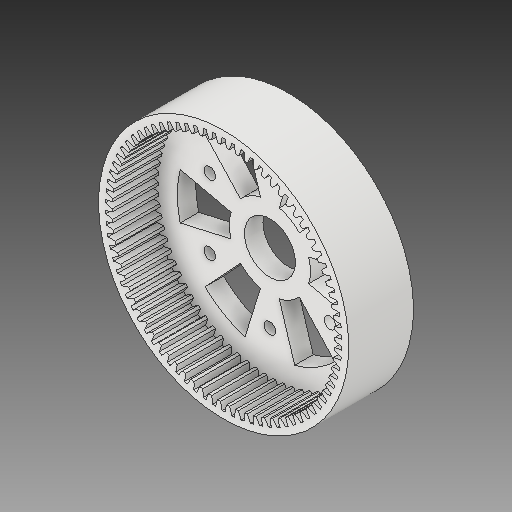
# Autodesk Inventor part: Basespline
Saved by Autodesk Inventor 2017 (Build 210142000, 142)
## iProperties
Created: 2017-07-11
Part Number: Basespline
Material: ABS Plastic
Document SubType Name: Modeling
Designer: zallen
Density: 1.06 g/cm^3
Appearance: CR White
Author: zallen
Autodesk Inventor part; units mm, degrees
ref_plane "YZ Plane" through (0, 0, 0) normal (1, 0, 0) x (0, 1, 0)
ref_plane "XZ Plane" through (0, 0, 0) normal (0, 1, 0) x (-1, 0, 0)
ref_plane "XY Plane" through (0, 0, 0) normal (0, 0, 1) x (1, 0, 0)
sketch "Sketch1" plane through (0, 0, 0) normal (0, 0, 1) x (1, 0, 0)
  circle A0 centre (0, 0) radius 45 construction
  circle A1 centre (0, 0) radius 48 construction
  circle A2 centre (0, 0) radius 48.1 construction
  circle A3 centre (0, 0) radius 51.1
  line L0 (0, 0) -> (73.8871, 0) construction
  circle A4 centre (0, 0) radius 54
  arc A5 (48.0963, -0.6) -> (51.0808, -1.4) centre (53.4515, 13.4115) ccw
  arc A6 (48.0963, 0.6) -> (48.0963, -0.6) centre (68.0873, 0) ccw
  arc A7 (51.0808, 1.4) -> (48.0963, 0.6) centre (53.4515, -13.4115) ccw
  arc A8 (51.0808, -1.4) -> (51.0808, 1.4) centre (0, 0) ccw
  circle A9 centre (0, 0) radius 51.1
  arc A10 (47.9886, 3.2721) -> (51.0278, 2.7148) centre (52.199, 17.669) ccw
  arc A11 (50.8025, 5.5058) -> (47.892, 4.4682) centre (54.3573, -9.0669) ccw
  arc A12 (51.0278, 2.7148) -> (50.8025, 5.5058) centre (0, 0) ccw
  arc A13 (47.892, 4.4682) -> (47.9886, 3.2721) centre (67.8665, 5.4787) ccw
  circle A14 centre (0, 0) radius 51.1
  arc A15 (47.5697, 7.123) -> (50.6439, 6.8121) centre (50.6079, 21.812) ccw
  arc A16 (50.1948, 9.5758) -> (47.3772, 8.3074) centre (54.9107, -4.6636) ccw
  arc A17 (50.6439, 6.8121) -> (50.1948, 9.5758) centre (0, 0) ccw
  arc A18 (47.3772, 8.3074) -> (47.5697, 7.123) centre (67.2055, 10.922) ccw
  circle A19 centre (0, 0) radius 51.1
  arc A20 (46.8423, 10.9276) -> (49.9315, 10.8651) centre (48.6887, 25.8135) ccw
  arc A21 (49.2615, 13.5838) -> (46.5551, 12.0928) centre (55.1079, -0.23) ccw
  arc A22 (49.9315, 10.8651) -> (49.2615, 13.5838) centre (0, 0) ccw
  arc A23 (46.5551, 12.0928) -> (46.8423, 10.9276) centre (66.1088, 16.2943) ccw
  circle A24 centre (0, 0) radius 51.1
  arc A25 (45.8111, 14.6614) -> (48.8954, 14.8477) centre (46.4537, 29.6477) ccw
  arc A26 (48.0087, 17.5036) -> (45.4311, 15.7997) centre (54.9477, 4.2051) ccw
  arc A27 (48.8954, 14.8477) -> (48.0087, 17.5036) centre (0, 0) ccw
  arc A28 (45.4311, 15.7997) -> (45.8111, 14.6614) centre (64.5832, 21.5611) ccw
  circle A29 centre (0, 0) radius 51.1
  arc A30 (44.4827, 18.3001) -> (47.5421, 18.734) centre (43.9174, 33.2895) ccw
  arc A31 (46.4445, 21.3099) -> (44.0124, 19.4041) centre (54.4311, 8.6129) ccw
  arc A32 (47.5421, 18.734) -> (46.4445, 21.3099) centre (0, 0) ccw
  arc A33 (44.0124, 19.4041) -> (44.4827, 18.3001) centre (62.6389, 26.6879) ccw
  circle A34 centre (0, 0) radius 51.1
  arc A35 (42.866, 21.8202) -> (45.8804, 22.4988) centre (41.0963, 36.7154) ccw
  arc A36 (44.5792, 24.9781) -> (42.3083, 22.8827) centre (53.5616, 12.9649) ccw
  arc A37 (45.8804, 22.4988) -> (44.5792, 24.9781) centre (0, 0) ccw
  arc A38 (42.3083, 22.8827) -> (42.866, 21.8202) centre (60.2883, 31.6417) ccw
  circle A39 centre (0, 0) radius 51.1
  arc A40 (40.9712, 25.1987) -> (43.9213, 26.1177) centre (38.0087, 39.9032) ccw
  arc A41 (42.4247, 28.4842) -> (40.3298, 26.2129) centre (52.3446, 17.2327) ccw
  arc A42 (43.9213, 26.1177) -> (42.4247, 28.4842) centre (0, 0) ccw
  arc A43 (40.3298, 26.2129) -> (40.9712, 25.1987) centre (57.5467, 36.3903) ccw
  circle A44 centre (0, 0) radius 51.1
  arc A45 (38.8107, 28.4138) -> (41.6772, 29.5672) centre (34.6746, 42.8323) ccw
  arc A46 (39.9952, 31.8056) -> (38.0898, 29.3731) centre (50.7882, 21.3889) ccw
  arc A47 (41.6772, 29.5672) -> (39.9952, 31.8056) centre (0, 0) ccw
  arc A48 (38.0898, 29.3731) -> (38.8107, 28.4138) centre (54.4319, 40.9029) ccw
  circle A49 centre (0, 0) radius 51.1
  arc A50 (36.3984, 31.4446) -> (39.1629, 32.8249) centre (31.1156, 45.4835) ccw
  arc A51 (37.3062, 34.9208) -> (35.6027, 32.3428) centre (48.9025, 25.4062) ccw
  arc A52 (39.1629, 32.8249) -> (37.3062, 34.9208) centre (0, 0) ccw
  arc A53 (35.6027, 32.3428) -> (36.3984, 31.4446) centre (50.964, 45.1502) ccw
  circle A54 centre (0, 0) radius 51.1
  arc A55 (33.7502, 34.2715) -> (36.3946, 35.8698) centre (27.3547, 47.8398) ccw
  arc A56 (34.3752, 37.8094) -> (32.8847, 35.1028) centre (46.6995, 29.2589) ccw
  arc A57 (36.3946, 35.8698) -> (34.3752, 37.8094) centre (0, 0) ccw
  arc A58 (32.8847, 35.1028) -> (33.7502, 34.2715) centre (47.1657, 49.1047) ccw
  circle A59 centre (0, 0) radius 51.1
  arc A60 (30.883, 36.8761) -> (33.3903, 38.682) centre (23.4165, 49.8858) ccw
  arc A61 (31.2214, 40.4529) -> (29.9535, 37.6351) centre (44.1937, 32.9218) ccw
  arc A62 (33.3903, 38.682) -> (31.2214, 40.4529) centre (0, 0) ccw
  arc A63 (29.9535, 37.6351) -> (30.883, 36.8761) centre (43.0615, 52.7407) ccw
  circle A64 centre (0, 0) radius 51.1
  arc A65 (27.8156, 39.2416) -> (30.1694, 41.2434) centre (19.3265, 51.6083) ccw
  arc A66 (27.865, 42.834) -> (26.828, 39.9233) centre (41.4013, 36.3711) ccw
  arc A67 (30.1694, 41.2434) -> (27.865, 42.834) centre (0, 0) ccw
  arc A68 (26.828, 39.9233) -> (27.8156, 39.2416) centre (38.678, 56.0347) ccw
  circle A69 centre (0, 0) radius 51.1
  arc A70 (24.5677, 41.3526) -> (26.7528, 43.5373) centre (15.1111, 52.9961) ccw
  arc A71 (24.328, 44.9373) -> (23.5285, 41.9526) centre (38.3404, 39.5846) ccw
  arc A72 (26.7528, 43.5373) -> (24.328, 44.9373) centre (0, 0) ccw
  arc A73 (23.5285, 41.9526) -> (24.5677, 41.3526) centre (34.0436, 58.9653) ccw
  circle A74 centre (0, 0) radius 51.1
  arc A75 (21.1606, 43.1954) -> (23.1628, 45.5488) centre (10.7976, 54.0402) ccw
  arc A76 (20.6331, 46.7492) -> (20.0764, 43.7098) centre (35.0309, 42.5414) ccw
  arc A77 (23.1628, 45.5488) -> (20.6331, 46.7492) centre (0, 0) ccw
  arc A78 (20.0764, 43.7098) -> (21.1606, 43.1954) centre (29.1885, 61.5135) ccw
  circle A79 centre (0, 0) radius 51.1
  arc A80 (17.6162, 44.758) -> (19.4225, 47.2649) centre (6.4142, 54.7338) ccw
  arc A81 (16.8045, 48.2578) -> (16.4942, 45.1835) centre (31.4941, 45.2222) ccw
  arc A82 (19.4225, 47.2649) -> (16.8045, 48.2578) centre (0, 0) ccw
  arc A83 (16.4942, 45.1835) -> (17.6162, 44.758) centre (24.1441, 63.6627) ccw
  circle A84 centre (0, 0) radius 51.1
  arc A85 (13.9575, 46.0304) -> (15.5563, 48.6745) centre (1.9892, 55.0724) ccw
  arc A86 (12.8669, 49.4536) -> (12.8049, 46.3643) centre (27.7531, 47.6098) ccw
  arc A87 (15.5563, 48.6745) -> (12.8669, 49.4536) centre (0, 0) ccw
  arc A88 (12.8049, 46.3643) -> (13.9575, 46.0304) centre (18.9431, 65.399) ccw
  circle A89 centre (0, 0) radius 51.1
  arc A90 (10.2084, 47.0042) -> (11.5892, 49.7685) centre (-2.4488, 55.0539) ccw
  arc A91 (8.8458, 50.3285) -> (9.0326, 47.2443) centre (23.8321, 49.6886) ccw
  arc A92 (11.5892, 49.7685) -> (8.8458, 50.3285) centre (0, 0) ccw
  arc A93 (9.0326, 47.2443) -> (10.2084, 47.0042) centre (13.6192, 66.7113) ccw
  circle A94 centre (0, 0) radius 51.1
  arc A95 (6.393, 47.6733) -> (7.5469, 50.5396) centre (-6.8708, 54.6783) ccw
  arc A96 (4.7673, 50.8771) -> (5.2017, 47.8179) centre (19.7566, 51.4452) ccw
  arc A97 (7.5469, 50.5396) -> (4.7673, 50.8771) centre (0, 0) ccw
  arc A98 (5.2017, 47.8179) -> (6.393, 47.6733) centre (8.207, 67.5908) ccw
  circle A99 centre (0, 0) radius 51.1
  arc A100 (2.5362, 48.0331) -> (3.4557, 50.983) centre (-11.2483, 53.9482) ccw
  arc A101 (0.658, 51.0958) -> (1.3371, 48.0814) centre (15.5529, 52.8681) ccw
  arc A102 (3.4557, 50.983) -> (0.658, 51.0958) centre (0, 0) ccw
  arc A103 (1.3371, 48.0814) -> (2.5362, 48.0331) centre (2.7416, 68.032) ccw
  circle A104 centre (0, 0) radius 51.1
  arc A105 (-1.3371, 48.0814) -> (-0.658, 51.0958) centre (-15.5529, 52.8681) ccw
  arc A106 (-3.4557, 50.983) -> (-2.5362, 48.0331) centre (11.2483, 53.9482) ccw
  arc A107 (-0.658, 51.0958) -> (-3.4557, 50.983) centre (0, 0) ccw
  arc A108 (-2.5362, 48.0331) -> (-1.3371, 48.0814) centre (-2.7416, 68.032) ccw
  circle A109 centre (0, 0) radius 51.1
  arc A110 (-5.2017, 47.8179) -> (-4.7673, 50.8771) centre (-19.7566, 51.4452) ccw
  arc A111 (-7.5469, 50.5396) -> (-6.393, 47.6733) centre (6.8708, 54.6783) ccw
  arc A112 (-4.7673, 50.8771) -> (-7.5469, 50.5396) centre (0, 0) ccw
  arc A113 (-6.393, 47.6733) -> (-5.2017, 47.8179) centre (-8.207, 67.5908) ccw
  circle A114 centre (0, 0) radius 51.1
  arc A115 (-9.0326, 47.2443) -> (-8.8458, 50.3285) centre (-23.8321, 49.6886) ccw
  arc A116 (-11.5892, 49.7685) -> (-10.2084, 47.0042) centre (2.4488, 55.0539) ccw
  arc A117 (-8.8458, 50.3285) -> (-11.5892, 49.7685) centre (0, 0) ccw
  arc A118 (-10.2084, 47.0042) -> (-9.0326, 47.2443) centre (-13.6192, 66.7113) ccw
  circle A119 centre (0, 0) radius 51.1
  arc A120 (-12.8049, 46.3643) -> (-12.8669, 49.4536) centre (-27.7531, 47.6098) ccw
  arc A121 (-15.5563, 48.6745) -> (-13.9575, 46.0304) centre (-1.9892, 55.0724) ccw
  arc A122 (-12.8669, 49.4536) -> (-15.5563, 48.6745) centre (0, 0) ccw
  arc A123 (-13.9575, 46.0304) -> (-12.8049, 46.3643) centre (-18.9431, 65.399) ccw
  circle A124 centre (0, 0) radius 51.1
  arc A125 (-16.4942, 45.1835) -> (-16.8045, 48.2578) centre (-31.4941, 45.2222) ccw
  arc A126 (-19.4225, 47.2649) -> (-17.6162, 44.758) centre (-6.4142, 54.7338) ccw
  arc A127 (-16.8045, 48.2578) -> (-19.4225, 47.2649) centre (0, 0) ccw
  arc A128 (-17.6162, 44.758) -> (-16.4942, 45.1835) centre (-24.1441, 63.6627) ccw
  circle A129 centre (0, 0) radius 51.1
  arc A130 (-20.0764, 43.7098) -> (-20.6331, 46.7492) centre (-35.0309, 42.5414) ccw
  arc A131 (-23.1628, 45.5488) -> (-21.1606, 43.1954) centre (-10.7976, 54.0402) ccw
  arc A132 (-20.6331, 46.7492) -> (-23.1628, 45.5488) centre (0, 0) ccw
  arc A133 (-21.1606, 43.1954) -> (-20.0764, 43.7098) centre (-29.1885, 61.5135) ccw
  circle A134 centre (0, 0) radius 51.1
  arc A135 (-23.5285, 41.9526) -> (-24.328, 44.9373) centre (-38.3404, 39.5846) ccw
  arc A136 (-26.7528, 43.5373) -> (-24.5677, 41.3526) centre (-15.1111, 52.9961) ccw
  arc A137 (-24.328, 44.9373) -> (-26.7528, 43.5373) centre (0, 0) ccw
  arc A138 (-24.5677, 41.3526) -> (-23.5285, 41.9526) centre (-34.0436, 58.9653) ccw
  circle A139 centre (0, 0) radius 51.1
  arc A140 (-26.828, 39.9233) -> (-27.865, 42.834) centre (-41.4013, 36.3711) ccw
  arc A141 (-30.1694, 41.2434) -> (-27.8156, 39.2416) centre (-19.3265, 51.6083) ccw
  arc A142 (-27.865, 42.834) -> (-30.1694, 41.2434) centre (0, 0) ccw
  arc A143 (-27.8156, 39.2416) -> (-26.828, 39.9233) centre (-38.678, 56.0347) ccw
  circle A144 centre (0, 0) radius 51.1
  arc A145 (-29.9535, 37.6351) -> (-31.2214, 40.4529) centre (-44.1937, 32.9218) ccw
  arc A146 (-33.3903, 38.682) -> (-30.883, 36.8761) centre (-23.4165, 49.8858) ccw
  arc A147 (-31.2214, 40.4529) -> (-33.3903, 38.682) centre (0, 0) ccw
  arc A148 (-30.883, 36.8761) -> (-29.9535, 37.6351) centre (-43.0615, 52.7407) ccw
  circle A149 centre (0, 0) radius 51.1
  arc A150 (-32.8847, 35.1028) -> (-34.3752, 37.8094) centre (-46.6995, 29.2589) ccw
  arc A151 (-36.3946, 35.8698) -> (-33.7502, 34.2715) centre (-27.3547, 47.8398) ccw
  arc A152 (-34.3752, 37.8094) -> (-36.3946, 35.8698) centre (0, 0) ccw
  arc A153 (-33.7502, 34.2715) -> (-32.8847, 35.1028) centre (-47.1657, 49.1047) ccw
  circle A154 centre (0, 0) radius 51.1
  arc A155 (-35.6027, 32.3428) -> (-37.3062, 34.9208) centre (-48.9025, 25.4062) ccw
  arc A156 (-39.1629, 32.8249) -> (-36.3984, 31.4446) centre (-31.1156, 45.4835) ccw
  arc A157 (-37.3062, 34.9208) -> (-39.1629, 32.8249) centre (0, 0) ccw
  arc A158 (-36.3984, 31.4446) -> (-35.6027, 32.3428) centre (-50.964, 45.1502) ccw
  circle A159 centre (0, 0) radius 51.1
  arc A160 (-38.0898, 29.3731) -> (-39.9952, 31.8056) centre (-50.7882, 21.3889) ccw
  arc A161 (-41.6772, 29.5672) -> (-38.8107, 28.4138) centre (-34.6746, 42.8323) ccw
  arc A162 (-39.9952, 31.8056) -> (-41.6772, 29.5672) centre (0, 0) ccw
  arc A163 (-38.8107, 28.4138) -> (-38.0898, 29.3731) centre (-54.4319, 40.9029) ccw
  circle A164 centre (0, 0) radius 51.1
  arc A165 (-40.3298, 26.2129) -> (-42.4247, 28.4842) centre (-52.3446, 17.2327) ccw
  arc A166 (-43.9213, 26.1177) -> (-40.9712, 25.1987) centre (-38.0087, 39.9032) ccw
  arc A167 (-42.4247, 28.4842) -> (-43.9213, 26.1177) centre (0, 0) ccw
  arc A168 (-40.9712, 25.1987) -> (-40.3298, 26.2129) centre (-57.5467, 36.3903) ccw
  circle A169 centre (0, 0) radius 51.1
  arc A170 (-42.3083, 22.8827) -> (-44.5792, 24.9781) centre (-53.5616, 12.9649) ccw
  arc A171 (-45.8804, 22.4988) -> (-42.866, 21.8202) centre (-41.0963, 36.7154) ccw
  arc A172 (-44.5792, 24.9781) -> (-45.8804, 22.4988) centre (0, 0) ccw
  arc A173 (-42.866, 21.8202) -> (-42.3083, 22.8827) centre (-60.2883, 31.6417) ccw
  circle A174 centre (0, 0) radius 51.1
  arc A175 (-44.0124, 19.4041) -> (-46.4445, 21.3099) centre (-54.4311, 8.6129) ccw
  arc A176 (-47.5421, 18.734) -> (-44.4827, 18.3001) centre (-43.9174, 33.2895) ccw
  arc A177 (-46.4445, 21.3099) -> (-47.5421, 18.734) centre (0, 0) ccw
  arc A178 (-44.4827, 18.3001) -> (-44.0124, 19.4041) centre (-62.6389, 26.6879) ccw
  circle A179 centre (0, 0) radius 51.1
  arc A180 (-45.4311, 15.7997) -> (-48.0087, 17.5036) centre (-54.9477, 4.2051) ccw
  arc A181 (-48.8954, 14.8477) -> (-45.8111, 14.6614) centre (-46.4537, 29.6477) ccw
  arc A182 (-48.0087, 17.5036) -> (-48.8954, 14.8477) centre (0, 0) ccw
  arc A183 (-45.8111, 14.6614) -> (-45.4311, 15.7997) centre (-64.5832, 21.5611) ccw
  circle A184 centre (0, 0) radius 51.1
  arc A185 (-46.5551, 12.0928) -> (-49.2615, 13.5838) centre (-55.1079, -0.23) ccw
  arc A186 (-49.9315, 10.8651) -> (-46.8423, 10.9276) centre (-48.6887, 25.8135) ccw
  arc A187 (-49.2615, 13.5838) -> (-49.9315, 10.8651) centre (0, 0) ccw
  arc A188 (-46.8423, 10.9276) -> (-46.5551, 12.0928) centre (-66.1088, 16.2943) ccw
  circle A189 centre (0, 0) radius 51.1
  arc A190 (-47.3772, 8.3074) -> (-50.1948, 9.5758) centre (-54.9107, -4.6636) ccw
  arc A191 (-50.6439, 6.8121) -> (-47.5697, 7.123) centre (-50.6079, 21.812) ccw
  arc A192 (-50.1948, 9.5758) -> (-50.6439, 6.8121) centre (0, 0) ccw
  arc A193 (-47.5697, 7.123) -> (-47.3772, 8.3074) centre (-67.2055, 10.922) ccw
  circle A194 centre (0, 0) radius 51.1
  arc A195 (-47.892, 4.4682) -> (-50.8025, 5.5058) centre (-54.3573, -9.0669) ccw
  arc A196 (-51.0278, 2.7148) -> (-47.9886, 3.2721) centre (-52.199, 17.669) ccw
  arc A197 (-50.8025, 5.5058) -> (-51.0278, 2.7148) centre (0, 0) ccw
  arc A198 (-47.9886, 3.2721) -> (-47.892, 4.4682) centre (-67.8665, 5.4787) ccw
  circle A199 centre (0, 0) radius 51.1
  arc A200 (-48.0963, 0.6) -> (-51.0808, 1.4) centre (-53.4515, -13.4115) ccw
  arc A201 (-51.0808, -1.4) -> (-48.0963, -0.6) centre (-53.4515, 13.4115) ccw
  arc A202 (-51.0808, 1.4) -> (-51.0808, -1.4) centre (0, 0) ccw
  arc A203 (-48.0963, -0.6) -> (-48.0963, 0.6) centre (-68.0873, 0) ccw
  circle A204 centre (0, 0) radius 51.1
  arc A205 (-47.9886, -3.2721) -> (-51.0278, -2.7148) centre (-52.199, -17.669) ccw
  arc A206 (-50.8025, -5.5058) -> (-47.892, -4.4682) centre (-54.3573, 9.0669) ccw
  arc A207 (-51.0278, -2.7148) -> (-50.8025, -5.5058) centre (0, 0) ccw
  arc A208 (-47.892, -4.4682) -> (-47.9886, -3.2721) centre (-67.8665, -5.4787) ccw
  circle A209 centre (0, 0) radius 51.1
  arc A210 (-47.5697, -7.123) -> (-50.6439, -6.8121) centre (-50.6079, -21.812) ccw
  arc A211 (-50.1948, -9.5758) -> (-47.3772, -8.3074) centre (-54.9107, 4.6636) ccw
  arc A212 (-50.6439, -6.8121) -> (-50.1948, -9.5758) centre (0, 0) ccw
  arc A213 (-47.3772, -8.3074) -> (-47.5697, -7.123) centre (-67.2055, -10.922) ccw
  circle A214 centre (0, 0) radius 51.1
  arc A215 (-46.8423, -10.9276) -> (-49.9315, -10.8651) centre (-48.6887, -25.8135) ccw
  arc A216 (-49.2615, -13.5838) -> (-46.5551, -12.0928) centre (-55.1079, 0.23) ccw
  arc A217 (-49.9315, -10.8651) -> (-49.2615, -13.5838) centre (0, 0) ccw
  arc A218 (-46.5551, -12.0928) -> (-46.8423, -10.9276) centre (-66.1088, -16.2943) ccw
  circle A219 centre (0, 0) radius 51.1
  arc A220 (-45.8111, -14.6614) -> (-48.8954, -14.8477) centre (-46.4537, -29.6477) ccw
  arc A221 (-48.0087, -17.5036) -> (-45.4311, -15.7997) centre (-54.9477, -4.2051) ccw
  arc A222 (-48.8954, -14.8477) -> (-48.0087, -17.5036) centre (0, 0) ccw
  arc A223 (-45.4311, -15.7997) -> (-45.8111, -14.6614) centre (-64.5832, -21.5611) ccw
  circle A224 centre (0, 0) radius 51.1
  arc A225 (-44.4827, -18.3001) -> (-47.5421, -18.734) centre (-43.9174, -33.2895) ccw
  arc A226 (-46.4445, -21.3099) -> (-44.0124, -19.4041) centre (-54.4311, -8.6129) ccw
  arc A227 (-47.5421, -18.734) -> (-46.4445, -21.3099) centre (0, 0) ccw
  arc A228 (-44.0124, -19.4041) -> (-44.4827, -18.3001) centre (-62.6389, -26.6879) ccw
  circle A229 centre (0, 0) radius 51.1
  arc A230 (-42.866, -21.8202) -> (-45.8804, -22.4988) centre (-41.0963, -36.7154) ccw
  arc A231 (-44.5792, -24.9781) -> (-42.3083, -22.8827) centre (-53.5616, -12.9649) ccw
  arc A232 (-45.8804, -22.4988) -> (-44.5792, -24.9781) centre (0, 0) ccw
  arc A233 (-42.3083, -22.8827) -> (-42.866, -21.8202) centre (-60.2883, -31.6417) ccw
  circle A234 centre (0, 0) radius 51.1
  arc A235 (-40.9712, -25.1987) -> (-43.9213, -26.1177) centre (-38.0087, -39.9032) ccw
  arc A236 (-42.4247, -28.4842) -> (-40.3298, -26.2129) centre (-52.3446, -17.2327) ccw
  arc A237 (-43.9213, -26.1177) -> (-42.4247, -28.4842) centre (0, 0) ccw
  arc A238 (-40.3298, -26.2129) -> (-40.9712, -25.1987) centre (-57.5467, -36.3903) ccw
  circle A239 centre (0, 0) radius 51.1
  arc A240 (-38.8107, -28.4138) -> (-41.6772, -29.5672) centre (-34.6746, -42.8323) ccw
  arc A241 (-39.9952, -31.8056) -> (-38.0898, -29.3731) centre (-50.7882, -21.3889) ccw
  arc A242 (-41.6772, -29.5672) -> (-39.9952, -31.8056) centre (0, 0) ccw
  arc A243 (-38.0898, -29.3731) -> (-38.8107, -28.4138) centre (-54.4319, -40.9029) ccw
  circle A244 centre (0, 0) radius 51.1
  arc A245 (-36.3984, -31.4446) -> (-39.1629, -32.8249) centre (-31.1156, -45.4835) ccw
  arc A246 (-37.3062, -34.9208) -> (-35.6027, -32.3428) centre (-48.9025, -25.4062) ccw
  arc A247 (-39.1629, -32.8249) -> (-37.3062, -34.9208) centre (0, 0) ccw
  arc A248 (-35.6027, -32.3428) -> (-36.3984, -31.4446) centre (-50.964, -45.1502) ccw
  circle A249 centre (0, 0) radius 51.1
  arc A250 (-33.7502, -34.2715) -> (-36.3946, -35.8698) centre (-27.3547, -47.8398) ccw
  arc A251 (-34.3752, -37.8094) -> (-32.8847, -35.1028) centre (-46.6995, -29.2589) ccw
  arc A252 (-36.3946, -35.8698) -> (-34.3752, -37.8094) centre (0, 0) ccw
  arc A253 (-32.8847, -35.1028) -> (-33.7502, -34.2715) centre (-47.1657, -49.1047) ccw
  circle A254 centre (0, 0) radius 51.1
  arc A255 (-30.883, -36.8761) -> (-33.3903, -38.682) centre (-23.4165, -49.8858) ccw
  arc A256 (-31.2214, -40.4529) -> (-29.9535, -37.6351) centre (-44.1937, -32.9218) ccw
  arc A257 (-33.3903, -38.682) -> (-31.2214, -40.4529) centre (0, 0) ccw
  arc A258 (-29.9535, -37.6351) -> (-30.883, -36.8761) centre (-43.0615, -52.7407) ccw
  circle A259 centre (0, 0) radius 51.1
  arc A260 (-27.8156, -39.2416) -> (-30.1694, -41.2434) centre (-19.3265, -51.6083) ccw
  arc A261 (-27.865, -42.834) -> (-26.828, -39.9233) centre (-41.4013, -36.3711) ccw
  arc A262 (-30.1694, -41.2434) -> (-27.865, -42.834) centre (0, 0) ccw
  arc A263 (-26.828, -39.9233) -> (-27.8156, -39.2416) centre (-38.678, -56.0347) ccw
  circle A264 centre (0, 0) radius 51.1
  arc A265 (-24.5677, -41.3526) -> (-26.7528, -43.5373) centre (-15.1111, -52.9961) ccw
  arc A266 (-24.328, -44.9373) -> (-23.5285, -41.9526) centre (-38.3404, -39.5846) ccw
  arc A267 (-26.7528, -43.5373) -> (-24.328, -44.9373) centre (0, 0) ccw
  arc A268 (-23.5285, -41.9526) -> (-24.5677, -41.3526) centre (-34.0436, -58.9653) ccw
  circle A269 centre (0, 0) radius 51.1
  arc A270 (-21.1606, -43.1954) -> (-23.1628, -45.5488) centre (-10.7976, -54.0402) ccw
  arc A271 (-20.6331, -46.7492) -> (-20.0764, -43.7098) centre (-35.0309, -42.5414) ccw
  arc A272 (-23.1628, -45.5488) -> (-20.6331, -46.7492) centre (0, 0) ccw
  arc A273 (-20.0764, -43.7098) -> (-21.1606, -43.1954) centre (-29.1885, -61.5135) ccw
  circle A274 centre (0, 0) radius 51.1
  arc A275 (-17.6162, -44.758) -> (-19.4225, -47.2649) centre (-6.4142, -54.7338) ccw
  arc A276 (-16.8045, -48.2578) -> (-16.4942, -45.1835) centre (-31.4941, -45.2222) ccw
  arc A277 (-19.4225, -47.2649) -> (-16.8045, -48.2578) centre (0, 0) ccw
  arc A278 (-16.4942, -45.1835) -> (-17.6162, -44.758) centre (-24.1441, -63.6627) ccw
  circle A279 centre (0, 0) radius 51.1
  arc A280 (-13.9575, -46.0304) -> (-15.5563, -48.6745) centre (-1.9892, -55.0724) ccw
  arc A281 (-12.8669, -49.4536) -> (-12.8049, -46.3643) centre (-27.7531, -47.6098) ccw
  arc A282 (-15.5563, -48.6745) -> (-12.8669, -49.4536) centre (0, 0) ccw
  arc A283 (-12.8049, -46.3643) -> (-13.9575, -46.0304) centre (-18.9431, -65.399) ccw
  circle A284 centre (0, 0) radius 51.1
  arc A285 (-10.2084, -47.0042) -> (-11.5892, -49.7685) centre (2.4488, -55.0539) ccw
  arc A286 (-8.8458, -50.3285) -> (-9.0326, -47.2443) centre (-23.8321, -49.6886) ccw
  arc A287 (-11.5892, -49.7685) -> (-8.8458, -50.3285) centre (0, 0) ccw
  arc A288 (-9.0326, -47.2443) -> (-10.2084, -47.0042) centre (-13.6192, -66.7113) ccw
  circle A289 centre (0, 0) radius 51.1
  arc A290 (-6.393, -47.6733) -> (-7.5469, -50.5396) centre (6.8708, -54.6783) ccw
  arc A291 (-4.7673, -50.8771) -> (-5.2017, -47.8179) centre (-19.7566, -51.4452) ccw
  arc A292 (-7.5469, -50.5396) -> (-4.7673, -50.8771) centre (0, 0) ccw
  arc A293 (-5.2017, -47.8179) -> (-6.393, -47.6733) centre (-8.207, -67.5908) ccw
  circle A294 centre (0, 0) radius 51.1
  arc A295 (-2.5362, -48.0331) -> (-3.4557, -50.983) centre (11.2483, -53.9482) ccw
  arc A296 (-0.658, -51.0958) -> (-1.3371, -48.0814) centre (-15.5529, -52.8681) ccw
  arc A297 (-3.4557, -50.983) -> (-0.658, -51.0958) centre (0, 0) ccw
  arc A298 (-1.3371, -48.0814) -> (-2.5362, -48.0331) centre (-2.7416, -68.032) ccw
  circle A299 centre (0, 0) radius 51.1
  arc A300 (1.3371, -48.0814) -> (0.658, -51.0958) centre (15.5529, -52.8681) ccw
  arc A301 (3.4557, -50.983) -> (2.5362, -48.0331) centre (-11.2483, -53.9482) ccw
  arc A302 (0.658, -51.0958) -> (3.4557, -50.983) centre (0, 0) ccw
  arc A303 (2.5362, -48.0331) -> (1.3371, -48.0814) centre (2.7416, -68.032) ccw
  circle A304 centre (0, 0) radius 51.1
  arc A305 (5.2017, -47.8179) -> (4.7673, -50.8771) centre (19.7566, -51.4452) ccw
  arc A306 (7.5469, -50.5396) -> (6.393, -47.6733) centre (-6.8708, -54.6783) ccw
  arc A307 (4.7673, -50.8771) -> (7.5469, -50.5396) centre (0, 0) ccw
  arc A308 (6.393, -47.6733) -> (5.2017, -47.8179) centre (8.207, -67.5908) ccw
  circle A309 centre (0, 0) radius 51.1
  arc A310 (9.0326, -47.2443) -> (8.8458, -50.3285) centre (23.8321, -49.6886) ccw
  arc A311 (11.5892, -49.7685) -> (10.2084, -47.0042) centre (-2.4488, -55.0539) ccw
  arc A312 (8.8458, -50.3285) -> (11.5892, -49.7685) centre (0, 0) ccw
  arc A313 (10.2084, -47.0042) -> (9.0326, -47.2443) centre (13.6192, -66.7113) ccw
  circle A314 centre (0, 0) radius 51.1
  arc A315 (12.8049, -46.3643) -> (12.8669, -49.4536) centre (27.7531, -47.6098) ccw
  arc A316 (15.5563, -48.6745) -> (13.9575, -46.0304) centre (1.9892, -55.0724) ccw
  arc A317 (12.8669, -49.4536) -> (15.5563, -48.6745) centre (0, 0) ccw
  arc A318 (13.9575, -46.0304) -> (12.8049, -46.3643) centre (18.9431, -65.399) ccw
  circle A319 centre (0, 0) radius 51.1
  arc A320 (16.4942, -45.1835) -> (16.8045, -48.2578) centre (31.4941, -45.2222) ccw
  arc A321 (19.4225, -47.2649) -> (17.6162, -44.758) centre (6.4142, -54.7338) ccw
  arc A322 (16.8045, -48.2578) -> (19.4225, -47.2649) centre (0, 0) ccw
  arc A323 (17.6162, -44.758) -> (16.4942, -45.1835) centre (24.1441, -63.6627) ccw
  circle A324 centre (0, 0) radius 51.1
  arc A325 (20.0764, -43.7098) -> (20.6331, -46.7492) centre (35.0309, -42.5414) ccw
  arc A326 (23.1628, -45.5488) -> (21.1606, -43.1954) centre (10.7976, -54.0402) ccw
  arc A327 (20.6331, -46.7492) -> (23.1628, -45.5488) centre (0, 0) ccw
  arc A328 (21.1606, -43.1954) -> (20.0764, -43.7098) centre (29.1885, -61.5135) ccw
  circle A329 centre (0, 0) radius 51.1
  arc A330 (23.5285, -41.9526) -> (24.328, -44.9373) centre (38.3404, -39.5846) ccw
  arc A331 (26.7528, -43.5373) -> (24.5677, -41.3526) centre (15.1111, -52.9961) ccw
  arc A332 (24.328, -44.9373) -> (26.7528, -43.5373) centre (0, 0) ccw
  arc A333 (24.5677, -41.3526) -> (23.5285, -41.9526) centre (34.0436, -58.9653) ccw
  circle A334 centre (0, 0) radius 51.1
  arc A335 (26.828, -39.9233) -> (27.865, -42.834) centre (41.4013, -36.3711) ccw
  arc A336 (30.1694, -41.2434) -> (27.8156, -39.2416) centre (19.3265, -51.6083) ccw
  arc A337 (27.865, -42.834) -> (30.1694, -41.2434) centre (0, 0) ccw
  arc A338 (27.8156, -39.2416) -> (26.828, -39.9233) centre (38.678, -56.0347) ccw
  circle A339 centre (0, 0) radius 51.1
  arc A340 (29.9535, -37.6351) -> (31.2214, -40.4529) centre (44.1937, -32.9218) ccw
  arc A341 (33.3903, -38.682) -> (30.883, -36.8761) centre (23.4165, -49.8858) ccw
  arc A342 (31.2214, -40.4529) -> (33.3903, -38.682) centre (0, 0) ccw
  arc A343 (30.883, -36.8761) -> (29.9535, -37.6351) centre (43.0615, -52.7407) ccw
  circle A344 centre (0, 0) radius 51.1
  arc A345 (32.8847, -35.1028) -> (34.3752, -37.8094) centre (46.6995, -29.2589) ccw
  arc A346 (36.3946, -35.8698) -> (33.7502, -34.2715) centre (27.3547, -47.8398) ccw
  arc A347 (34.3752, -37.8094) -> (36.3946, -35.8698) centre (0, 0) ccw
  arc A348 (33.7502, -34.2715) -> (32.8847, -35.1028) centre (47.1657, -49.1047) ccw
  circle A349 centre (0, 0) radius 51.1
  arc A350 (35.6027, -32.3428) -> (37.3062, -34.9208) centre (48.9025, -25.4062) ccw
  arc A351 (39.1629, -32.8249) -> (36.3984, -31.4446) centre (31.1156, -45.4835) ccw
  arc A352 (37.3062, -34.9208) -> (39.1629, -32.8249) centre (0, 0) ccw
  arc A353 (36.3984, -31.4446) -> (35.6027, -32.3428) centre (50.964, -45.1502) ccw
  circle A354 centre (0, 0) radius 51.1
  arc A355 (38.0898, -29.3731) -> (39.9952, -31.8056) centre (50.7882, -21.3889) ccw
  arc A356 (41.6772, -29.5672) -> (38.8107, -28.4138) centre (34.6746, -42.8323) ccw
  arc A357 (39.9952, -31.8056) -> (41.6772, -29.5672) centre (0, 0) ccw
  arc A358 (38.8107, -28.4138) -> (38.0898, -29.3731) centre (54.4319, -40.9029) ccw
  circle A359 centre (0, 0) radius 51.1
  arc A360 (40.3298, -26.2129) -> (42.4247, -28.4842) centre (52.3446, -17.2327) ccw
  arc A361 (43.9213, -26.1177) -> (40.9712, -25.1987) centre (38.0087, -39.9032) ccw
  arc A362 (42.4247, -28.4842) -> (43.9213, -26.1177) centre (0, 0) ccw
  arc A363 (40.9712, -25.1987) -> (40.3298, -26.2129) centre (57.5467, -36.3903) ccw
  circle A364 centre (0, 0) radius 51.1
  arc A365 (42.3083, -22.8827) -> (44.5792, -24.9781) centre (53.5616, -12.9649) ccw
  arc A366 (45.8804, -22.4988) -> (42.866, -21.8202) centre (41.0963, -36.7154) ccw
  arc A367 (44.5792, -24.9781) -> (45.8804, -22.4988) centre (0, 0) ccw
  arc A368 (42.866, -21.8202) -> (42.3083, -22.8827) centre (60.2883, -31.6417) ccw
  circle A369 centre (0, 0) radius 51.1
  arc A370 (44.0124, -19.4041) -> (46.4445, -21.3099) centre (54.4311, -8.6129) ccw
  arc A371 (47.5421, -18.734) -> (44.4827, -18.3001) centre (43.9174, -33.2895) ccw
  arc A372 (46.4445, -21.3099) -> (47.5421, -18.734) centre (0, 0) ccw
  arc A373 (44.4827, -18.3001) -> (44.0124, -19.4041) centre (62.6389, -26.6879) ccw
  circle A374 centre (0, 0) radius 51.1
  arc A375 (45.4311, -15.7997) -> (48.0087, -17.5036) centre (54.9477, -4.2051) ccw
  arc A376 (48.8954, -14.8477) -> (45.8111, -14.6614) centre (46.4537, -29.6477) ccw
  arc A377 (48.0087, -17.5036) -> (48.8954, -14.8477) centre (0, 0) ccw
  arc A378 (45.8111, -14.6614) -> (45.4311, -15.7997) centre (64.5832, -21.5611) ccw
  circle A379 centre (0, 0) radius 51.1
  arc A380 (46.5551, -12.0928) -> (49.2615, -13.5838) centre (55.1079, 0.23) ccw
  arc A381 (49.9315, -10.8651) -> (46.8423, -10.9276) centre (48.6887, -25.8135) ccw
  arc A382 (49.2615, -13.5838) -> (49.9315, -10.8651) centre (0, 0) ccw
  arc A383 (46.8423, -10.9276) -> (46.5551, -12.0928) centre (66.1088, -16.2943) ccw
  circle A384 centre (0, 0) radius 51.1
  arc A385 (47.3772, -8.3074) -> (50.1948, -9.5758) centre (54.9107, 4.6636) ccw
  arc A386 (50.6439, -6.8121) -> (47.5697, -7.123) centre (50.6079, -21.812) ccw
  arc A387 (50.1948, -9.5758) -> (50.6439, -6.8121) centre (0, 0) ccw
  arc A388 (47.5697, -7.123) -> (47.3772, -8.3074) centre (67.2055, -10.922) ccw
  circle A389 centre (0, 0) radius 51.1
  arc A390 (47.892, -4.4682) -> (50.8025, -5.5058) centre (54.3573, 9.0669) ccw
  arc A391 (51.0278, -2.7148) -> (47.9886, -3.2721) centre (52.199, -17.669) ccw
  arc A392 (50.8025, -5.5058) -> (51.0278, -2.7148) centre (0, 0) ccw
  arc A393 (47.9886, -3.2721) -> (47.892, -4.4682) centre (67.8665, -5.4787) ccw
  point P0 (48.0873, 0)
  point P1 (47.9313, 3.8694)
  point P2 (47.4645, 7.7137)
  point P3 (46.6899, 11.508)
  point P4 (45.6125, 15.2277)
  point P5 (44.2393, 18.8486)
  point P6 (42.5792, 22.3473)
  point P7 (40.6429, 25.701)
  point P8 (38.443, 28.888)
  point P9 (35.9938, 31.8877)
  point P10 (33.3112, 34.6806)
  point P11 (30.4126, 37.2486)
  point P12 (27.3167, 39.575)
  point P13 (24.0436, 41.6448)
  point P14 (20.6146, 43.4445)
  point P15 (17.052, 44.9624)
  point P16 (13.3787, 46.1887)
  point P17 (9.6187, 47.1154)
  point P18 (5.7963, 47.7366)
  point P19 (1.9363, 48.0483)
  point P20 (-1.9363, 48.0483)
  point P21 (-5.7963, 47.7366)
  point P22 (-9.6187, 47.1154)
  point P23 (-13.3787, 46.1887)
  point P24 (-17.052, 44.9624)
  point P25 (-20.6146, 43.4445)
  point P26 (-24.0436, 41.6448)
  point P27 (-27.3167, 39.575)
  point P28 (-30.4126, 37.2486)
  point P29 (-33.3112, 34.6806)
  point P30 (-35.9938, 31.8877)
  point P31 (-38.443, 28.888)
  point P32 (-40.6429, 25.701)
  point P33 (-42.5792, 22.3473)
  point P34 (-44.2393, 18.8486)
  point P35 (-45.6125, 15.2277)
  point P36 (-46.6899, 11.508)
  point P37 (-47.4645, 7.7137)
  point P38 (-47.9313, 3.8694)
  point P39 (-48.0873, 0)
  point P40 (-47.9313, -3.8694)
  point P41 (-47.4645, -7.7137)
  point P42 (-46.6899, -11.508)
  point P43 (-45.6125, -15.2277)
  point P44 (-44.2393, -18.8486)
  point P45 (-42.5792, -22.3473)
  point P46 (-40.6429, -25.701)
  point P47 (-38.443, -28.888)
  point P48 (-35.9938, -31.8877)
  point P49 (-33.3112, -34.6806)
  point P50 (-30.4126, -37.2486)
  point P51 (-27.3167, -39.575)
  point P52 (-24.0436, -41.6448)
  point P53 (-20.6146, -43.4445)
  point P54 (-17.052, -44.9624)
  point P55 (-13.3787, -46.1887)
  point P56 (-9.6187, -47.1154)
  point P57 (-5.7963, -47.7366)
  point P58 (-1.9363, -48.0483)
  point P59 (1.9363, -48.0483)
  point P60 (5.7963, -47.7366)
  point P61 (9.6187, -47.1154)
  point P62 (13.3787, -46.1887)
  point P63 (17.052, -44.9624)
  point P64 (20.6146, -43.4445)
  point P65 (24.0436, -41.6448)
  point P66 (27.3167, -39.575)
  point P67 (30.4126, -37.2486)
  point P68 (33.3112, -34.6806)
  point P69 (35.9938, -31.8877)
  point P70 (38.443, -28.888)
  point P71 (40.6429, -25.701)
  point P72 (42.5792, -22.3473)
  point P73 (44.2393, -18.8486)
  point P74 (45.6125, -15.2277)
  point P75 (46.6899, -11.508)
  point P76 (47.4645, -7.7137)
  point P77 (47.9313, -3.8694)
  dimension "d0" = 90
  dimension "d1" = 3
  dimension "d2" = 0.1
  dimension "d3" = 3
  dimension "d4" = 108
  dimension "d5" = 15
  dimension "d6" = 20
  dimension "d7" = 1.2
  dimension "d8" = 1.4
  dimension "d15" = 360
  constraints: 627 point on circle, 316 centre point, 4 coincident, 2 end point, 2 symmetric about line, 1 horizontal, 1 point on line, 1482 other
  measures "d0" diameter of A0
  measures "d1" radial gap between concentric circles of A0 A1
  measures "d2" radial gap between concentric circles of A1 A2
  measures "d4" diameter of A4
  measures "d5" radius of A5
  measures "d6" radius of A6
  measures "d7" distance of A2.end A2.start
  measures "d8" distance from line of L0 A5.end
extrude "Extrusion1" add sketch "Sketch1" along normal blind 20 contours A3 A5 A6 A7 | A10 A13 A11 A3 | A3 A390 A393 A391 | A15 A18 A16 A3 | A3 A385 A388 A386 | A20 A23 A21 A3 | A3 A380 A383 A381 | A25 A28 A26 A3 | A3 A375 A378 A376 | A30 A33 A31 A3 | A3 A370 A373 A371 | A35 A38 A36 A3 | A3 A365 A368 A366 | A40 A43 A41 A3 | A3 A360 A363 A361 | A45 A48 A46 A3 | A3 A355 A358 A356 | A50 A53 A51 A3 | A3 A350 A353 A351 | A55 A58 A56 A3 | A3 A345 A348 A346 | A60 A63 A61 A3 | A3 A340 A343 A341 | A65 A68 A66 A3 | A3 A335 A338 A336 | A70 A73 A71 A3 | A3 A330 A333 A331 | A75 A78 A76 A3 | A3 A325 A328 A326 | A80 A83 A81 A3 | A3 A320 A323 A321 | A85 A88 A86 A3 | A3 A315 A318 A316 | A90 A93 A91 A3 | A3 A310 A313 A311 | A95 A98 A96 A3 | A3 A305 A308 A306 | A100 A103 A101 A3 | A3 A300 A303 A301 | A105 A108 A106 A3 | A3 A295 A298 A296 | A110 A113 A111 A3 | A3 A290 A293 A291 | A115 A118 A116 A3 | A3 A285 A288 A286 | A120 A123 A121 A3 | A3 A280 A283 A281 | A125 A128 A126 A3 | A3 A275 A278 A276 | A130 A133 A131 A3 | A3 A270 A273 A271 | A135 A138 A136 A3 | A3 A265 A268 A266 | A140 A143 A141 A3 | A3 A260 A263 A261 | A145 A148 A146 A3 | A3 A255 A258 A256 | A150 A153 A151 A3 | A3 A250 A253 A251 | A155 A158 A156 A3 | A3 A245 A248 A246 | A160 A163 A161 A3 | A3 A240 A243 A241 | A165 A168 A166 A3 | A3 A235 A238 A236 | A170 A173 A171 A3 | A3 A230 A233 A231 | A175 A178 A176 A3 | A3 A225 A228 A226 | A180 A183 A181 A3 | A3 A220 A223 A221 | A185 A188 A186 A3 | A3 A215 A218 A216 | A190 A193 A191 A3 | A3 A210 A213 A211 | A195 A198 A196 A3 | A3 A205 A208 A206 | A200 A203 A201 A3 | A4
sketch "Sketch2" plane through (0, 0, 0) normal (0, 0, -1) x (-1, 0, 0)
  circle A0 centre (0, 0) radius 54 projected
  circle A1 centre (0, 0) radius 11
  circle A2 centre (0, 0) radius 40 construction
  line L0 (38.7298, 10) -> (16.7705, 5)
  line L1 (38.7298, -10) -> (16.7705, -5)
  arc A3 (16.7705, -5) -> (16.7705, 5) centre (0, 0) ccw
  arc A4 (38.7298, -10) -> (38.7298, 10) centre (0, 0) ccw
  circle A5 centre (0, 0) radius 17.5 construction
  line L2 (10.7047, 38.541) -> (4.0551, 17.0237)
  arc A6 (12.7154, 12.0237) -> (4.0551, 17.0237) centre (0, 0) ccw
  line L3 (28.0252, 28.541) -> (12.7154, 12.0237)
  circle A7 centre (0, 0) radius 40 construction
  arc A8 (28.0252, 28.541) -> (10.7047, 38.541) centre (0, 0) ccw
  line L4 (-28.0252, 28.541) -> (-12.7154, 12.0237)
  arc A9 (-4.0551, 17.0237) -> (-12.7154, 12.0237) centre (0, 0) ccw
  line L5 (-10.7047, 38.541) -> (-4.0551, 17.0237)
  circle A10 centre (0, 0) radius 40 construction
  arc A11 (-10.7047, 38.541) -> (-28.0252, 28.541) centre (0, 0) ccw
  line L6 (-38.7298, -10) -> (-16.7705, -5)
  arc A12 (-16.7705, 5) -> (-16.7705, -5) centre (0, 0) ccw
  line L7 (-38.7298, 10) -> (-16.7705, 5)
  circle A13 centre (0, 0) radius 40 construction
  arc A14 (-38.7298, 10) -> (-38.7298, -10) centre (0, 0) ccw
  line L8 (-10.7047, -38.541) -> (-4.0551, -17.0237)
  arc A15 (-12.7154, -12.0237) -> (-4.0551, -17.0237) centre (0, 0) ccw
  line L9 (-28.0252, -28.541) -> (-12.7154, -12.0237)
  circle A16 centre (0, 0) radius 40 construction
  arc A17 (-28.0252, -28.541) -> (-10.7047, -38.541) centre (0, 0) ccw
  line L10 (28.0252, -28.541) -> (12.7154, -12.0237)
  arc A18 (4.0551, -17.0237) -> (12.7154, -12.0237) centre (0, 0) ccw
  line L11 (10.7047, -38.541) -> (4.0551, -17.0237)
  circle A19 centre (0, 0) radius 40 construction
  arc A20 (10.7047, -38.541) -> (28.0252, -28.541) centre (0, 0) ccw
  circle A21 centre (0, 0) radius 30 construction
  circle A22 centre (25.9808, -15) radius 2.5
  line L12 (28.974, -7.7787) -> (21.2235, -21.2029) construction
  line L13 (25.0988, -14.4908) -> (25.9808, -15) construction
  circle A23 centre (25.9808, 15) radius 2.5
  circle A24 centre (0, 30) radius 2.5
  circle A25 centre (-25.9808, 15) radius 2.5
  circle A26 centre (-25.9808, -15) radius 2.5
  circle A27 centre (0, -30) radius 2.5
  point P0 (17.5, 0)
  point P1 (40, 0)
  point P2 (8.75, 15.1554)
  point P3 (20, 34.641)
  point P4 (-8.75, 15.1554)
  point P5 (-20, 34.641)
  point P6 (-17.5, 0)
  point P7 (-40, 0)
  point P8 (-8.75, -15.1554)
  point P9 (-20, -34.641)
  point P10 (8.75, -15.1554)
  point P11 (20, -34.641)
  dimension "d21" = 80
  dimension "d35" = 35
  dimension "d19" = 22
  dimension "d22" = 10
  dimension "d23" = 5
  dimension "d32" = 10
  dimension "d33" = 5
  dimension "d42" = 360
  dimension "d46" = 60
  dimension "d47" = 5
  dimension "d48" = 90
  dimension "d51" = 360
  constraints: 29 point on circle, 28 end point, 20 centre point, 10 coincident, 2 point on line, 1 midpoint, 126 other
  measures "d19" diameter of A1
  measures "d22" vertical distance of point (0, 0) L0.start
  measures "d23" vertical distance of point (0, 0) L0.end
  measures "d32" vertical distance of L1.start point (40, 0)
  measures "d33" vertical distance of point (0, 0) L1.end
  measures "d46" diameter of A21
  measures "d47" diameter of A22
  measures "d48" angle of L12 L13
extrude "Extrusion2" add sketch "Sketch2" along normal blind 8
body "Solid1"
